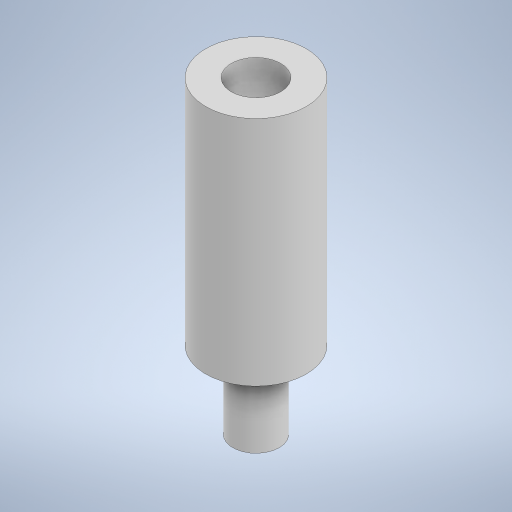
# Autodesk Inventor part: ControlPanel_shortStands
Saved by Autodesk Inventor 2024.2 (Build 282272000, 272)
## iProperties
Created: 2024-04-16
Part Number: ControlPanel_shortStands
Material: Generic
Document SubType Name: Modeling
Designer: ringl
Density: 1 g/cm^3
Appearance: Default
Author: ringl
Autodesk Inventor part; units mm, degrees
ref_plane "YZ Plane" through (0, 0, 0) normal (1, 0, 0) x (0, 1, 0)
ref_plane "XZ Plane" through (0, 0, 0) normal (0, 1, 0) x (-1, 0, 0)
ref_plane "XY Plane" through (0, 0, 0) normal (0, 0, 1) x (1, 0, 0)
sketch "Sketch1" plane through (0, 0, 0) normal (0, 1, 0) x (-1, 0, 0)
  circle A0 centre (0, 0) radius 1.5
  dimension "d0" = 3
  constraints: 1 centre point, 1 coincident
  measures "d0" diameter of A0
extrude "Extrusion1" add sketch "Sketch1" along normal blind 5
sketch "Sketch2" plane through (0, 5, 0) normal (0, 1, 0) x (1, 0, 0)
  circle A0 centre (0, 0) radius 1.5 projected
  circle A1 centre (0, 0) radius 3.25
  dimension "d3" = 6.5
  constraints: 1 centre point, 1 coincident
  measures "d3" diameter of A1
extrude "Extrusion2" add sketch "Sketch2" along normal blind 15 contours A0 | A1
sketch "Sketch3" plane through (0, 20, 0) normal (0, 1, 0) x (1, 0, 0)
  circle A0 centre (0, 0) radius 1.5 projected
  circle A1 centre (0, 0) radius 1.6
  dimension "d6" = 3.2
  constraints: 1 centre point, 1 coincident
  measures "d6" diameter of A1
extrude "Extrusion3" cut sketch "Sketch3" against normal blind 2.5 contours A0 | A1
body "Solid1"
